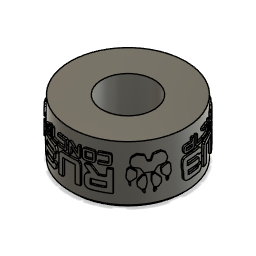
light v2 (Autodesk Fusion 360 design; units mm, degrees)
Autodesk Fusion 360 part; units mm, degrees
sketch "Esquisse1" plane through (0, 0, 0) normal (0, 1, 0) x (1, 0, 0)
  line L0 (25, 200) -> (-25, 200)
  line L1 (-25, 200) -> (-25, -200)
  line L2 (-25, -200) -> (25, -200)
  line L3 (25, -200) -> (25, 200)
  line L4 (25, 200) -> (-25, -200) construction
  line L5 (-25, 200) -> (25, -200) construction
  circle A0 centre (0, 100) radius 6.5
  circle A1 centre (0, 100) radius 4
  dimension "d1" = 50
  dimension "d2" = 400
  dimension "d3" = 13
  dimension "d4" = 8
  constraint horizontal L0
  constraint perpendicular L0 L1
  constraint parallel L0 L2
  constraint parallel L1 L3
  constraint coincident L4 origin
  constraint coincident L5 origin
  constraint concentric A0 A1
  measures "d1" distance of L1.end L2.end
  measures "d2" distance of L0.end L1.end
  measures "d3" diameter of A0
  measures "d4" diameter of A1
extrude "Extrusion1" add sketch "Esquisse1" against normal blind 6 contours L0 L1 L2 L3 makes body 1
extrude "Extrusion2" add sketch "Esquisse1" against normal blind 7 contours A0 bodies 1
fillet "Congé1" radius 3 1 edges at (-6.0601, -7, -102.3505) on bodies 1
extrude "Extrusion3" add 1 faces at (0.1619, -6, 102.1606) along direction (0, -1, 0) blind 9 and the other way blind -3 on bodies 1 bodies 1 makes body 2
extrude "Extrusion4" add sketch "Esquisse1" along normal blind -15 and the other way blind 8 contours A0 bodies 2
fillet "Congé2" radius 3 1 edges at (-6.0601, -8, -102.3505) on bodies 2
extrude "Extrusion5" add 1 faces at (0, -15, 101.3333) along direction (0, -1, 0) blind 6.5 and the other way blind -0.5 separate body on bodies 2 makes body 3
extrude "Extrusion6" add sketch "Esquisse1" along normal blind -22.5 and the other way blind 15.5 contours A0 bodies 3
fillet "Congé3" radius 3 1 edges at (-6.0601, -22.5, -102.3505) on bodies 3
extrude "Extrusion7" add sketch "Esquisse1" along normal blind 1 contours A0 bodies 1
fillet "Congé4" radius 3 1 edges at (-6.0601, 1, -97.6495) on bodies 1
extrude "Extrusion8" cut 2 faces at (-8.3333, -17.5, 200) (-8.3333, -11, 200) along direction (0, 0, -1) blind 270 on bodies 2 3 bodies 2 3
extrude "Extrusion9" add 1 faces at (-0.0996, -15, -167.9963) along direction (0, -1, 0) blind 0.25 separate body on bodies 2 makes body 4
revolve "Révolution1" add 1 faces at (-8.3333, -11, -70) angle 180 about axis through (25, -15.25, -70) along (1, 0, 0) on bodies 2 bodies 2 3 4
extrude "Extrusion10" cut 1 faces at (-0.0996, -15.25, -167.9963) along direction (0, 1, 0) blind 0.25 on bodies 2 bodies 2
sketch "Esquisse2" plane through (0, 0, 0) normal (0, -1, 0) x (1, 0, 0)
  line L0 (25, -70) -> (-25, -70)
  line L1 (-25, -70) -> (-25, -200)
  line L2 (-25, -200) -> (25, -200)
  line L3 (25, -200) -> (25, -70)
  circle A0 centre (0, -100) radius 6.5
  circle A1 centre (0, -100) radius 10
  circle A2 centre (0, -100) radius 3.5
  circle A3 centre (0, -100) radius 6.5
  line L4 (25, 200) -> (25, -200)
  line L5 (25, -200) -> (-25, -200)
  line L6 (-25, -200) -> (-25, 200)
  line L7 (-25, 200) -> (25, 200)
  dimension "d42" = 7
  constraint concentric A0 A1
  constraint concentric A1 A2
  measures "d42" diameter of A2
extrude "Extrusion11" add sketch "Esquisse2" along normal blind -1 and the other way blind 4 separate body contours A0 A3 | A1 | A2 makes body 5
fillet "Congé5" radius 2 1 edges at (-9.3233, 4, -96.3838) on bodies 5
fillet "Congé6" radius 1 1 edges at (-9.3233, 1, -96.3838) on bodies 5
extrude "Extrusion12" add sketch "Esquisse2" along normal blind 22.5 and the other way blind 1 contours A2 bodies 5
extrude "Extrusion13" add 1 faces at (1.7216, -22.5, -100.6592) along direction (0, -1, 0) blind 12 on bodies 5 bodies 5
ref_plane "Plan de construction1" through (0, 0, -100) normal (0, 0, 1) x (1, 0, 0)
sketch "Esquisse3" plane through (0, 0, -100) normal (0, 0, 1) x (1, 0, 0)
  line L0 (0, -32.5) -> (0, -22.5)
  line L1 (0, -22.5) -> (0, -22.7)
  circle A0 centre (0, -25.5) radius 1.7
  line L2 (0, -34.5) -> (-1.5, -34.5)
  line L3 (-1.5, -34.5) -> (-1.5, -32.5)
  circle A1 centre (-1.5, -32.5) radius 2
  circle A2 centre (1.5, -32.5) radius 2
  line L4 (3.5, -34.5) -> (3.5, -31.3)
  line L5 (-3.5, -34.5) -> (3.5, -34.5)
  line L6 (3.5, -34.5) -> (-3.5, -34.5)
  line L7 (-3.5, -34.5) -> (-3.5, -31.3)
  dimension "d60" = 3.4
  dimension "d65" = 1.5
  dimension "d66" = 2
  dimension "d67" = 4
  constraint vertical L0
  constraint coincident L0 L1.end
  constraint horizontal L2
  constraint perpendicular L2 L3
  constraint coincident L3.end A1.centre
  constraint symmetric L0 A1 A2
  constraint vertical L4
  constraint tangent A2 L4
  constraint coincident L4.start L5
  constraint coincident L4.start L5.end
  constraint coincident L5.start L6.end
  constraint perpendicular L6 L7
  constraint coincident L0 A0.centre
  measures "d60" diameter of A0
  measures "d65" distance of L2.start L2.end
  measures "d66" distance of L2.end L3.end
  measures "d67" diameter of A1
extrude "Extrusion14" cut sketch "Esquisse3" along normal blind 5 and the other way blind 5 contours L0 A0 | L0 A0 bodies 5
thread "Filetage2" "ISO Metric profile 7.0 M7x1 6g" major diameter 6.884 minor diameter 5.744 pitch 1 angle 60 modelled right hand crest width 0.1446 on face at (-2.0275, -19.6639, -102.8529) crest through (3.442, 1.25, -100) on bodies 5
revolve "Révolution2" cut sketch "Esquisse3" angle 360 about axis through (0, -32.5, -100) along (0, 1, 0) contours A1 L5 L6 L7 | A2 L4 L5 L6 bodies 5
sketch "Esquisse5" plane through (0, -34.5, 0) normal (0, -1, 0) x (1, 0, 0)
  circle A0 centre (0, -100) radius 1.5
  circle A1 centre (0, -100) radius 10
  circle A2 centre (0, -100) radius 3.5
  circle A3 centre (0, -100) radius 5.5
  circle A4 centre (0, -100) radius 9
  circle A5 centre (0, -100) radius 8.9
  line L0 (0, -108.9) -> (7.7076, -104.45)
  line L1 (7.7076, -104.45) -> (7.7076, -95.55)
  line L2 (7.7076, -95.55) -> (0, -91.1)
  line L3 (0, -91.1) -> (-7.7076, -95.55)
  line L4 (-7.7076, -95.55) -> (-7.7076, -104.45)
  line L5 (-7.7076, -104.45) -> (0, -108.9)
  line L6 (0, -109) -> (7.7942, -104.5)
  line L7 (7.7942, -104.5) -> (7.7942, -95.5)
  line L8 (7.7942, -95.5) -> (0, -91)
  line L9 (0, -91) -> (-7.7942, -95.5)
  line L10 (-7.7942, -95.5) -> (-7.7942, -104.5)
  line L11 (-7.7942, -104.5) -> (0, -109)
  point P0 (0, -100)
  point P1 (0, -100)
  dimension "d69" = 20
  dimension "d70" = 7
  dimension "d71" = 11
  dimension "d94" = -1
  dimension "d95" = -1.1
  constraint concentric A0 A1
  constraint concentric A1 A2
  constraint concentric A1 A3
  constraint coincident P1 P0
  constraint coincident A5 L0.start
  constraint coincident A4 L6.start
  measures "d69" diameter of A1
  measures "d70" diameter of A2
  measures "d71" diameter of A3
extrude "Extrusion16" add sketch "Esquisse5" against normal blind 7 separate body contours A2 | A3 | L0 L1 L2 L3 L4 L5 makes body 6
extrude "Extrusion19" add sketch "Esquisse5" against normal blind 7 separate body contours A0 | A1 | A2 | A3 | A4 A5 L7 | A4 A5 L8 | A5 L7 L8 | A4 A5 L6 | A5 L6 L7 | A4 A5 L9 | A5 L8 L9 | A5 L1 L7 | A5 L7 | A5 L8 | A5 L2 L8 | A5 L6 L11 | A4 A5 L11 | A5 L0 L6 | A5 L6 | A4 A5 L10 | A5 L9 L10 | A5 L9 | A5 L3 L9 | L0 L1 L2 L3 L4 L5 | A5 L10 L11 | A5 L5 L11 | A5 L11 | A5 L10 | A5 L4 L10 makes body 7
extrude "Extrusion18" add sketch "Esquisse5" along normal blind 3 contours A0 | A1 | A2 | A3 | A4 A5 L7 | A4 A5 L8 | A5 L7 L8 | A4 A5 L6 | A5 L6 L7 | A4 A5 L9 | A5 L8 L9 | A5 L1 L7 | A5 L7 | A5 L8 | A5 L2 L8 | A5 L6 L11 | A4 A5 L11 | A5 L0 L6 | A5 L6 | A4 A5 L10 | A5 L9 L10 | A5 L9 | A5 L3 L9 | L0 L1 L2 L3 L4 L5 | A5 L10 L11 | A5 L5 L11 | A5 L11 | A5 L10 | A5 L4 L10 bodies 7
chamfer "Chanfrein1" distance 0.5 angle 45 1 edges at (-9.3233, -37.5, -103.6162) on bodies 7
thread "Filetage4" "ISO Metric profile 7.0 M7x1 6H" major diameter 7.1472 minor diameter 6.0355 pitch 1 angle 60 modelled right hand crest width 0.2748 on face at (-1.3822, -29.8333, -99.4173) crest through (3.0178, -34.25, -100) on bodies 6
sketch "Esquisse8" plane through (0, -37.5, 0) normal (0, -1, 0) x (1, 0, 0)
  circle A0 centre (0, -100) radius 9.5
  line L0 (2.9064, -104.5301) -> (-0.138, -104.5283)
  line L1 (-0.1715, -103.4006) -> (6.1362, -103.4173)
  line L2 (-0.1498, -91.2683) -> (0.7478, -91.2683)
  line L3 (-3.1825, -104.5265) -> (-3.4574, -104.8217)
  line L4 (-7.2363, -105.0821) -> (-7.7542, -104.339)
  line L5 (0.7478, -91.2683) -> (1.3542, -92.1337)
  line L6 (3.194, -98.4202) -> (1.5775, -95.7423)
  line L7 (2.503, -93.8005) -> (3.0454, -94.6019)
  line L8 (1.5775, -95.7423) -> (-0.039, -93.0644)
  line L9 (-3.4574, -104.8217) -> (-3.7323, -105.1169)
  line L10 (-6.4792, -103.384) -> (-0.1715, -103.4006)
  line L11 (-3.3039, -98.1262) -> (-4.1512, -99.5305)
  line L12 (-4.8051, -98.2895) -> (-3.7281, -96.6567)
  line L13 (6.9426, -105.1148) -> (5.1818, -105.1148)
  line L14 (3.8431, -99.4978) -> (3.194, -98.4202)
  line L15 (4.2948, -97.9642) -> (5.5443, -99.857)
  line L16 (-0.138, -104.5283) -> (-3.1825, -104.5265)
  line L17 (1.3542, -92.1337) -> (1.9606, -92.9991)
  line L18 (7.9945, -103.5616) -> (7.4685, -104.3382)
  line L19 (-5.8821, -99.9224) -> (-4.8051, -98.2895)
  line L20 (3.0454, -94.6019) -> (3.0454, -95.3366)
  line L21 (-0.0703, -93.012) -> (-0.1016, -92.9596)
  line L22 (-0.1016, -92.9596) -> (-0.1579, -92.9794)
  line L23 (5.8501, -102.8229) -> (5.5109, -102.2816)
  line L24 (1.9606, -92.9991) -> (2.503, -93.8005)
  line L25 (-3.7323, -105.1169) -> (-5.4843, -105.0995)
  line L26 (3.0454, -95.3366) -> (3.0454, -96.0713)
  line L27 (-5.4843, -105.0995) -> (-7.2363, -105.0821)
  line L28 (6.7694, -101.7093) -> (7.9945, -103.5616)
  line L29 (3.0454, -96.0713) -> (4.2948, -97.9642)
  line L30 (-0.039, -93.0644) -> (-0.0703, -93.012)
  line L31 (5.1818, -105.1148) -> (3.4211, -105.1148)
  line L32 (-3.29, -95.244) -> (-3.29, -94.4979)
  line L33 (5.5443, -99.857) -> (6.7694, -101.7093)
  line L34 (4.852, -101.1633) -> (4.4923, -100.5755)
  line L35 (-3.29, -95.99) -> (-3.29, -95.244)
  line L36 (6.1894, -103.3641) -> (5.8501, -102.8229)
  line L37 (7.4685, -104.3382) -> (6.9426, -105.1148)
  line L38 (-4.1512, -99.5305) -> (-5.3152, -101.4572)
  line L39 (-8.2721, -103.5958) -> (-8.1528, -103.3919)
  line L40 (5.5109, -102.2816) -> (5.3614, -102.0164)
  line L41 (6.1628, -103.3907) -> (6.1894, -103.3641)
  line L42 (-1.3355, -94.8606) -> (-2.4567, -96.722)
  line L43 (-0.1579, -92.9794) -> (-0.2143, -92.9991)
  line L44 (4.4923, -100.5755) -> (3.8431, -99.4978)
  line L45 (-8.0335, -103.188) -> (-6.9578, -101.5552)
  line L46 (-3.7281, -96.6567) -> (-3.5091, -96.3234)
  line L47 (3.4211, -105.1148) -> (3.1638, -104.8224)
  line L48 (3.1638, -104.8224) -> (2.9064, -104.5301)
  line L49 (-1.0475, -91.2683) -> (-0.1498, -91.2683)
  line L50 (6.1362, -103.4173) -> (6.1628, -103.3907)
  line L51 (-2.4567, -96.722) -> (-3.3039, -98.1262)
  line L52 (-3.5091, -96.3234) -> (-3.29, -95.99)
  line L53 (5.3614, -102.0164) -> (5.2118, -101.7511)
  line L54 (-2.1687, -92.8831) -> (-1.0475, -91.2683)
  line L55 (-0.2143, -92.9991) -> (-1.3355, -94.8606)
  line L56 (5.2118, -101.7511) -> (4.852, -101.1633)
  line L57 (-5.3152, -101.4572) -> (-6.4792, -103.384)
  line L58 (-6.9578, -101.5552) -> (-5.8821, -99.9224)
  line L59 (-3.29, -94.4979) -> (-2.1687, -92.8831)
  line L60 (-8.1528, -103.3919) -> (-8.0335, -103.188)
  line L61 (-7.7542, -104.339) -> (-8.2721, -103.5958)
  line L62 (0.0351, -98.5913) -> (0.144, -98.2118)
  line L63 (0.144, -98.2118) -> (0.2529, -97.8323)
  line L64 (1.8612, -98.5508) -> (1.8237, -98.7141)
  line L65 (0.2892, -97.7909) -> (0.6713, -97.6996)
  line L66 (0.3736, -100.0203) -> (-0.1356, -100.0193)
  line L67 (1.1187, -97.6116) -> (1.184, -97.6149)
  line L68 (0.3736, -100.0203) -> (-0.1356, -100.0193)
  line L69 (1.4126, -97.776) -> (1.6412, -97.937)
  line L70 (1.6412, -97.937) -> (1.7512, -98.2439)
  line L71 (1.6412, -97.937) -> (1.7512, -98.2439)
  line L72 (1.1187, -97.6116) -> (1.184, -97.6149)
  line L73 (1.8612, -98.5508) -> (1.8237, -98.7141)
  line L74 (0.2711, -97.8116) -> (0.2892, -97.7909)
  line L75 (0.6288, -102.3571) -> (0.5003, -102.5113)
  line L76 (0.6713, -97.6996) -> (1.0533, -97.6084)
  line L77 (0.3697, -102.4533) -> (0.3675, -102.241)
  line L78 (-0.4833, -100.4515) -> (-0.4304, -100.8401)
  line L79 (0.3719, -102.6655) -> (0.3697, -102.4533)
  line L80 (0.2892, -97.7909) -> (0.6713, -97.6996)
  line L81 (-1.7781, -100.7657) -> (-2.0742, -101.0058)
  line L82 (2.239, -100.0641) -> (2.2789, -100.5812)
  line L83 (1.8237, -98.7141) -> (1.7861, -98.8773)
  line L84 (-1.9511, -99.1986) -> (-2.0658, -98.9726)
  line L85 (1.7512, -98.2439) -> (1.8612, -98.5508)
  line L86 (1.4698, -100.7535) -> (1.2055, -100.507)
  line L87 (0.1063, -100.8661) -> (0.1063, -100.4332)
  line L88 (-0.4916, -98.1974) -> (-0.3719, -98.5508)
  line L89 (0.144, -98.2118) -> (0.2529, -97.8323)
  line L90 (0.5003, -102.5113) -> (0.3719, -102.6655)
  line L91 (0.0351, -98.5913) -> (0.144, -98.2118)
  line L92 (-1.9511, -99.1986) -> (-2.0658, -98.9726)
  line L93 (-0.1684, -98.571) -> (0.0351, -98.5913)
  line L94 (1.7512, -98.2439) -> (1.8612, -98.5508)
  line L95 (1.8237, -98.7141) -> (1.7861, -98.8773)
  line L96 (-2.3363, -100.9674) -> (-2.4596, -100.7558)
  line L97 (1.4126, -97.776) -> (1.6412, -97.937)
  line L98 (-0.8457, -100.3469) -> (-0.7453, -100.3479)
  line L99 (-0.6113, -97.8441) -> (-0.4916, -98.1974)
  line L100 (-1.1347, -99.3697) -> (-1.2817, -99.3355)
  line L101 (1.184, -97.6149) -> (1.4126, -97.776)
  line L102 (-1.4649, -97.6044) -> (-1.0645, -97.6978)
  line L103 (-1.9781, -97.9284) -> (-1.7215, -97.7664)
  line L104 (-1.1347, -99.3697) -> (-1.2817, -99.3355)
  line L105 (1.0533, -97.6084) -> (1.1187, -97.6116)
  line L106 (-0.6642, -97.7912) -> (-0.6378, -97.8176)
  line L107 (-0.4506, -101.5917) -> (-0.5237, -101.9547)
  line L108 (-2.1144, -101.1307) -> (-2.1144, -101.3723)
  line L109 (-0.4916, -98.1974) -> (-0.3719, -98.5508)
  line L110 (1.184, -97.6149) -> (1.4126, -97.776)
  line L111 (0.2529, -97.8323) -> (0.2711, -97.8116)
  line L112 (-0.3719, -98.5508) -> (-0.1684, -98.571)
  line L113 (0.2529, -97.8323) -> (0.2711, -97.8116)
  line L114 (-2.1484, -98.4665) -> (-2.1161, -98.1863)
  line L115 (1.0533, -97.6084) -> (1.1187, -97.6116)
  line L116 (-0.3719, -98.5508) -> (-0.1684, -98.571)
  line L117 (0.6713, -97.6996) -> (1.0533, -97.6084)
  line L118 (0.2711, -97.8116) -> (0.2892, -97.7909)
  line L119 (0.4792, -100.2816) -> (0.8153, -100.6369)
  line L120 (-1.3091, -100.9021) -> (-1.0774, -100.6245)
  line L121 (-0.6378, -97.8176) -> (-0.6113, -97.8441)
  line L122 (-1.4649, -97.6044) -> (-1.0645, -97.6978)
  line L123 (-0.6378, -97.8176) -> (-0.6113, -97.8441)
  line L124 (-2.1806, -98.7467) -> (-2.1484, -98.4665)
  line L125 (-0.6448, -100.0183) -> (-0.7167, -99.9703)
  line L126 (-2.3245, -101.1307) -> (-2.2194, -101.1307)
  line L127 (0.6941, -99.4891) -> (0.5961, -99.6141)
  line L128 (0.439, -100.2816) -> (0.4591, -100.2816)
  line L129 (-2.49, -99.553) -> (-2.3552, -99.4275)
  line L130 (1.7341, -101) -> (1.4698, -100.7535)
  line L131 (-1.4202, -101.4208) -> (-1.4433, -101.1633)
  line L132 (0.4982, -102.241) -> (0.6288, -102.241)
  line L133 (0.7921, -99.364) -> (0.6941, -99.4891)
  line L134 (-2.2053, -100.9866) -> (-2.3363, -100.9674)
  line L135 (0.5961, -99.6141) -> (0.4849, -99.8172)
  line L136 (1.2055, -100.507) -> (1.1784, -100.1494)
  line L137 (0.2727, -100.3574) -> (0.439, -100.2816)
  line L138 (-2.1751, -101.5519) -> (-2.2357, -101.4899)
  line L139 (1.9111, -101.1287) -> (1.806, -101.1287)
  line L140 (1.806, -101.1287) -> (1.806, -101.3704)
  line L141 (2.2789, -100.5812) -> (2.1706, -100.7906)
  line L142 (-1.4686, -100.1537) -> (-1.482, -100.5256)
  line L143 (1.1784, -100.1494) -> (1.1513, -99.7917)
  line L144 (0.9777, -101.8241) -> (0.8042, -102.0517)
  line L145 (-1.798, -99.5418) -> (-1.4552, -99.7818)
  line L146 (-1.4286, -99.3013) -> (-1.6898, -99.25)
  line L147 (2.1706, -100.7906) -> (2.0623, -101)
  line L148 (1.1513, -100.9922) -> (1.1513, -101.2944)
  line L149 (0.1063, -100.4332) -> (0.2727, -100.3574)
  line L150 (-1.482, -100.5256) -> (-1.7781, -100.7657)
  line L151 (-0.1356, -100.0193) -> (-0.6448, -100.0183)
  line L152 (1.618, -99.2117) -> (1.205, -99.2879)
  line L153 (-0.7991, -102.1104) -> (-0.9784, -102.1104)
  line L154 (0.4849, -99.8172) -> (0.3736, -100.0203)
  line L155 (2.0834, -99.4592) -> (2.1992, -99.547)
  line L156 (1.9274, -101.4879) -> (1.9718, -101.3083)
  line L157 (-0.9617, -99.646) -> (-1.1347, -99.3697)
  line L158 (-1.4552, -99.7818) -> (-1.4686, -100.1537)
  line L159 (1.1513, -101.2944) -> (1.1513, -101.5966)
  line L160 (-2.2801, -101.3103) -> (-2.3245, -101.1307)
  line L161 (-2.1144, -101.614) -> (-2.1751, -101.5519)
  line L162 (1.806, -101.612) -> (1.8667, -101.55)
  line L163 (0.6941, -99.4891) -> (0.5961, -99.6141)
  line L164 (1.4772, -99.5795) -> (1.803, -99.3672)
  line L165 (2.1992, -99.547) -> (2.239, -100.0641)
  line L166 (-0.6122, -102.1757) -> (-0.6122, -102.4043)
  line L167 (-0.8029, -102.2364) -> (-0.7101, -102.1777)
  line L168 (-2.2204, -99.3019) -> (-2.1806, -99.3019)
  line L169 (-0.5718, -102.0325) -> (-0.6199, -102.1104)
  line L170 (-2.5828, -100.5441) -> (-2.5364, -100.0486)
  line L171 (-0.7851, -102.464) -> (-0.8957, -102.2952)
  line L172 (-0.6199, -102.1104) -> (-0.7991, -102.1104)
  line L173 (-1.4286, -99.3013) -> (-1.6898, -99.25)
  line L174 (0.3567, -102.0124) -> (0.2315, -101.6557)
  line L175 (1.618, -99.2117) -> (1.205, -99.2879)
  line L176 (-0.9784, -102.1104) -> (-1.1878, -101.8944)
  line L177 (0.2315, -101.6557) -> (0.1063, -101.299)
  line L178 (-2.1806, -99.3019) -> (-2.1408, -99.3019)
  line L179 (1.9718, -101.3083) -> (2.0161, -101.1287)
  line L180 (-0.6611, -102.1767) -> (-0.6122, -102.1757)
  line L181 (0.6288, -102.2991) -> (0.6288, -102.3571)
  line L182 (-1.2817, -99.3355) -> (-1.4286, -99.3013)
  line L183 (0.8042, -102.0517) -> (0.5804, -102.032)
  line L184 (0.3675, -102.241) -> (0.4982, -102.241)
  line L185 (-0.5237, -101.9547) -> (-0.5718, -102.0325)
  line L186 (-0.8957, -102.2952) -> (-0.8029, -102.2364)
  line L187 (1.8854, -99.3693) -> (1.9677, -99.3714)
  line L188 (-2.4596, -100.7558) -> (-2.5828, -100.5441)
  line L189 (-0.6122, -102.4043) -> (-0.6122, -102.6329)
  line L190 (-0.6433, -102.6329) -> (-0.6745, -102.6329)
  line L191 (-0.6122, -102.6329) -> (-0.6433, -102.6329)
  line L192 (-0.7101, -102.1777) -> (-0.6611, -102.1767)
  line L193 (-0.6745, -102.6329) -> (-0.7851, -102.464)
  line L194 (2.0623, -101) -> (1.8982, -101)
  line L195 (0.6288, -102.241) -> (0.6288, -102.2991)
  line L196 (-1.6898, -99.25) -> (-1.9511, -99.1986)
  line L197 (1.806, -101.3704) -> (1.806, -101.612)
  line L198 (0.5961, -99.6141) -> (0.4849, -99.8172)
  line L199 (-0.7167, -99.9703) -> (-0.7886, -99.9224)
  line L200 (-1.0774, -100.6245) -> (-0.8457, -100.3469)
  line L201 (0.4849, -99.8172) -> (0.3736, -100.0203)
  line L202 (1.1513, -99.7917) -> (1.4772, -99.5795)
  line L203 (-2.0658, -98.9726) -> (-2.1806, -98.7467)
  line L204 (-0.7886, -99.9224) -> (-0.9617, -99.646)
  line L205 (-1.2817, -99.3355) -> (-1.4286, -99.3013)
  line L206 (-1.7215, -97.7664) -> (-1.4649, -97.6044)
  line L207 (1.9677, -99.3714) -> (2.0834, -99.4592)
  line L208 (-2.1161, -98.1863) -> (-2.0471, -98.0573)
  line L209 (1.8982, -101) -> (1.7341, -101)
  line L210 (-1.6898, -99.25) -> (-1.9511, -99.1986)
  line L211 (-0.6448, -100.0183) -> (-0.7167, -99.9703)
  line L212 (-2.0471, -98.0573) -> (-1.9781, -97.9284)
  line L213 (0.7921, -99.364) -> (0.6941, -99.4891)
  line L214 (1.1513, -101.5966) -> (0.9777, -101.8241)
  line L215 (0.4591, -100.2816) -> (0.4792, -100.2816)
  line L216 (1.702, -99.0445) -> (1.618, -99.2117)
  line L217 (-2.2357, -101.4899) -> (-2.2801, -101.3103)
  line L218 (-2.0658, -98.9726) -> (-2.1806, -98.7467)
  line L219 (-2.0742, -101.0058) -> (-2.2053, -100.9866)
  line L220 (-0.4304, -100.8401) -> (-0.3776, -101.2286)
  line L221 (-2.5364, -100.0486) -> (-2.49, -99.553)
  line L222 (1.8667, -101.55) -> (1.9274, -101.4879)
  line L223 (1.7861, -98.8773) -> (1.702, -99.0445)
  line L224 (-0.1356, -100.0193) -> (-0.6448, -100.0183)
  line L225 (-2.1161, -98.1863) -> (-2.0471, -98.0573)
  line L226 (-1.4433, -101.1633) -> (-1.3762, -101.0327)
  line L227 (-0.9617, -99.646) -> (-1.1347, -99.3697)
  line L228 (-0.6113, -97.8441) -> (-0.4916, -98.1974)
  line L229 (-2.1484, -98.4665) -> (-2.1161, -98.1863)
  line L230 (-0.1684, -98.571) -> (0.0351, -98.5913)
  line L231 (0.8153, -100.6369) -> (1.1513, -100.9922)
  line L232 (1.7861, -98.8773) -> (1.702, -99.0445)
  line L233 (-2.1144, -101.3723) -> (-2.1144, -101.614)
  line L234 (-1.9781, -97.9284) -> (-1.7215, -97.7664)
  line L235 (-2.2194, -101.1307) -> (-2.1144, -101.1307)
  line L236 (-0.564, -100.4002) -> (-0.4833, -100.4515)
  line L237 (-1.0645, -97.6978) -> (-0.6642, -97.7912)
  line L238 (-2.0471, -98.0573) -> (-1.9781, -97.9284)
  line L239 (0.1063, -101.299) -> (0.1063, -100.8661)
  line L240 (-0.6642, -97.7912) -> (-0.6378, -97.8176)
  line L241 (-2.3552, -99.4275) -> (-2.2204, -99.3019)
  line L242 (1.702, -99.0445) -> (1.618, -99.2117)
  line L243 (-1.0645, -97.6978) -> (-0.6642, -97.7912)
  line L244 (-0.7453, -100.3479) -> (-0.6448, -100.3489)
  line L245 (-0.6448, -100.3489) -> (-0.564, -100.4002)
  line L246 (1.803, -99.3672) -> (1.8854, -99.3693)
  line L247 (-1.3971, -101.6784) -> (-1.4202, -101.4208)
  line L248 (1.205, -99.2879) -> (0.7921, -99.364)
  line L249 (-0.7886, -99.9224) -> (-0.9617, -99.646)
  line L250 (-0.3776, -101.2286) -> (-0.4506, -101.5917)
  line L251 (0.5804, -102.032) -> (0.3567, -102.0124)
  line L252 (-1.3762, -101.0327) -> (-1.3091, -100.9021)
  line L253 (2.0161, -101.1287) -> (1.9111, -101.1287)
  line L254 (-0.7167, -99.9703) -> (-0.7886, -99.9224)
  line L255 (-2.1806, -98.7467) -> (-2.1484, -98.4665)
  line L256 (-2.1408, -99.3019) -> (-1.798, -99.5418)
  line L257 (-1.1878, -101.8944) -> (-1.3971, -101.6784)
  line L258 (1.205, -99.2879) -> (0.7921, -99.364)
  line L259 (-1.7215, -97.7664) -> (-1.4649, -97.6044)
  circle A1 centre (0, -100) radius 9.5
emboss "Gravure en relief2" depth -0.4 profiles "Esquisse8" section 1 contours L0 L2 L3 L4 L5 L7 L9 L12 L13 L15 L16 L17 L18 L19 L20 L24 L25 L26 L27 L28 L29 L31 L32 L33 L35 L37 L39 L45 L46 L47 L48 L49 L52 L54 L58 L59 L60 L61 | L62 L63 L64 L65 L66 L67 L68 L69 L70 L71 L72 L73 L74 L76 L80 L83 L84 L85 L88 L89 L91 L92 L93 L94 L95 L97 L99 L100 L101 L102 L103 L104 L105 L106 L109 L110 L111 L112 L113 L114 L115 L116 L117 L118 L121 L122 L123 L124 L125 L127 L133 L135 L146 L151 L152 L154 L157 L163 L173 L175 L182 L196 L198 L199 L201 L203 L204 L205 L206 L208 L210 L211 L212 L213 L216 L218 L223 L224 L225 L227 L228 L229 L230 L232 L234 L237 L238 L240 L242 L243 L248 L249 L254 L255 L258 L259 | L75 L77 L79 L90 L132 L181 L184 L195 | L78 L98 L107 L120 L131 L153 L169 L172 L176 L185 L200 L220 L226 L236 L244 L245 L247 L250 L252 L257 | L81 L96 L129 L134 L142 L145 L150 L158 L168 L170 L178 L188 L219 L221 L241 L256 | L82 L86 L130 L136 L141 L143 L147 L155 L164 L165 L187 L194 L202 L207 L209 L246 | L87 L119 L128 L137 L144 L148 L149 L159 L174 L177 L183 L214 L215 L231 L239 L251 | L108 L126 L138 L160 L161 L217 L233 L235 | L139 L140 L156 L162 L179 L197 L222 L253 | L166 L167 L171 L180 L186 L189 L190 L191 L192 L193 onto face at (-0.0584, -37.5, -92.9045) on bodies 7 bodies 7
sketch "Esquisse9" plane through (0, 0, 0) normal (0, 0, 1) x (1, 0, 0)
  line L0 (12.0165, -32.6685) -> (11.985, -32.2529)
  line L1 (7.6146, -32.7116) -> (7.6686, -32.1358)
  line L2 (8.9249, -31.8259) -> (8.9093, -32.258)
  line L3 (9.633, -32.4825) -> (9.7498, -32.4836)
  line L4 (13.2174, -32.1538) -> (13.2638, -32.7547)
  line L5 (-5.2181, -32.6758) -> (-5.2181, -33.03)
  spline S0 degree 3 poles (4.9372, -29.2993) (5.6787, -29.2993) (5.6974, -29.3018) (5.8108, -29.4152) knots 0 0 0 0 1 1 1 1
  line L6 (-4.9914, -29.9028) -> (-4.3917, -29.8896)
  line L7 (-4.1792, -32.3216) -> (-5.2181, -32.3216)
  line L8 (0.775, -30.3182) -> (0.4252, -29.8967)
  line L9 (0.0238, -31.0995) -> (0.0238, -30.1994)
  line L10 (-5.3978, -30.4917) -> (-5.4121, -30.716)
  line L11 (-4.3917, -29.8896) -> (-4.3776, -29.5945)
  line L12 (2.4794, -30.1966) -> (2.4794, -30.716)
  spline S1 degree 3 poles (-5.6709, -30.9377) (-5.8268, -30.7563) (-5.8368, -30.2283) (-5.688, -30.0391) knots 0 0 0 0 1 1 1 1
  line L13 (-3.4944, -29.2993) -> (-3.3291, -29.2993)
  line L14 (-2.0541, -30.9081) -> (-2.0541, -30.716)
  spline S2 degree 3 poles (3.8127, -29.4606) (3.8318, -29.4888) (3.8478, -29.822) (3.8482, -30.2011) knots 0 0 0 0 1 1 1 1
  line L15 (-5.557, -31.0702) -> (-5.6709, -30.9377)
  line L16 (-4.1759, -29.2993) -> (-3.9882, -29.2993)
  line L17 (0.4015, -30.4835) -> (0.3779, -31.0702)
  line L18 (-1.0638, -35.2023) -> (-1.4427, -35.2023)
  line L19 (-2.9986, -33.4078) -> (-2.9986, -33.7856)
  spline S3 degree 3 poles (-2.8033, -31.0938) (-3.3464, -31.0938) (-3.424, -31.0835) (-3.5353, -30.996) knots 0 0 0 0 1 1 1 1
  line L20 (-3.6597, -29.2993) -> (-3.4944, -29.2993)
  line L21 (3.5183, -30.1966) -> (3.5183, -29.6771)
  line L22 (5.5489, -30.716) -> (5.5489, -30.1966)
  spline S4 degree 3 poles (3.8482, -30.2011) (3.8491, -31.0902) (3.8717, -31.064) (3.0842, -31.0861) knots 0 0 0 0 1 1 1 1
  line L23 (4.8642, -30.716) -> (5.5489, -30.716)
  line L24 (-5.4121, -30.716) -> (-4.8901, -30.716)
  line L25 (-5.2181, -33.03) -> (-4.1083, -33.03)
  line L26 (-1.8216, -35.2023) -> (-1.808, -33.6237)
  line L27 (-2.7624, -34.1634) -> (-2.3847, -34.1634)
  line L28 (-5.0764, -34.1161) -> (-5.0764, -34.4467)
  line L29 (-2.6465, -35.0155) -> (-2.8148, -35.1787)
  line L30 (-3.1402, -34.4467) -> (-3.1402, -34.305)
  spline S5 degree 3 poles (5.8108, -29.4152) (5.9228, -29.5273) (5.9267, -29.553) (5.9252, -30.1826) knots 0 0 0 0 1 1 1 1
  line L31 (0.2008, -31.0849) -> (0.0238, -31.0995)
  spline S6 degree 3 poles (-5.688, -30.0391) (-5.5939, -29.9195) (-5.5743, -29.9157) (-4.9914, -29.9028) knots 0 0 0 0 1 1 1 1
  line L32 (4.1794, -30.716) -> (4.8642, -30.716)
  line L33 (6.0684, -35.2023) -> (4.4934, -35.2023)
  spline S7 degree 3 poles (-0.4312, -29.3972) (-0.3068, -29.4951) (-0.3068, -29.4953) (-0.3068, -30.1927) knots 0 0 0 0 1 1 1 1
  line L34 (-2.0541, -29.4882) -> (-2.0541, -29.2993)
  line L35 (-2.1958, -30.9049) -> (-2.1958, -31.0938)
  line L36 (-5.0764, -34.4467) -> (-4.1083, -34.4467)
  line L37 (-4.8757, -30.254) -> (-5.3834, -30.2674)
  line L38 (-4.3635, -29.2993) -> (-4.1759, -29.2993)
  spline S8 degree 3 poles (-5.8319, -34.1116) (-5.832, -33.6644) (-5.8506, -33.4796) (-5.9066, -33.3672) knots 0 0 0 0 1 1 1 1
  line L39 (-2.3847, -34.1634) -> (-2.385, -34.3404)
  line L40 (-1.4427, -35.2023) -> (-1.8216, -35.2023)
  spline S9 degree 3 poles (-5.4901, -35.1093) (-5.7801, -34.9302) (-5.8317, -34.7796) (-5.8319, -34.1116) knots 0 0 0 0 1 1 1 1
  spline S10 degree 3 poles (-5.8523, -31.8645) (-5.6448, -31.582) (-5.5559, -31.5662) (-4.1744, -31.5661) knots 0 0 0 0 1 1 1 1
  line L41 (4.2267, -33.5494) -> (3.1877, -33.5494)
  line L42 (-3.3291, -29.2993) -> (-3.3291, -30.0077)
  line L43 (-2.0541, -29.6771) -> (-2.0541, -29.4882)
  line L44 (-4.3776, -29.5945) -> (-4.3635, -29.2993)
  line L45 (4.2284, -32.7939) -> (4.7249, -32.7939)
  line L46 (-4.368, -30.4783) -> (-4.368, -30.2406)
  line L47 (-3.5353, -30.996) -> (-3.6597, -30.8981)
  line L48 (3.5183, -30.716) -> (3.5183, -30.1966)
  line L49 (1.4301, -29.9005) -> (1.4433, -29.2993)
  line L50 (-1.0513, -33.7738) -> (-1.0638, -35.2023)
  spline S11 degree 3 poles (1.6153, -31.0938) (1.4394, -31.0938) (1.3515, -31.0127) (0.775, -30.3182) knots 0 0 0 0 1 1 1 1
  line L51 (5.2892, -31.5897) -> (5.6788, -31.5759)
  line L52 (-4.7854, -31.0702) -> (-5.557, -31.0702)
  spline S12 degree 3 poles (4.7249, -32.7939) (5.1119, -32.7939) (5.227, -32.779) (5.2473, -32.7263) knots 0 0 0 0 1 1 1 1
  line L53 (3.5183, -29.6771) -> (2.9989, -29.6771)
  line L54 (3.1877, -34.4467) -> (4.2267, -34.4467)
  line L55 (-3.6597, -30.8981) -> (-3.6597, -30.0987)
  line L56 (4.1794, -30.9049) -> (4.1794, -30.716)
  spline S13 degree 3 poles (3.6836, -29.3558) (3.7355, -29.3852) (3.7937, -29.4324) (3.8127, -29.4606) knots 0 0 0 0 1 1 1 1
  line L57 (-4.001, -30.1848) -> (-4.0139, -31.0702)
  line L58 (-2.0541, -31.1002) -> (-2.0541, -30.9081)
  line L59 (4.1794, -29.4882) -> (4.1794, -29.2993)
  line L60 (0.3779, -31.0702) -> (0.2008, -31.0849)
  line L61 (4.1794, -29.6771) -> (4.1794, -29.4882)
  spline S14 degree 3 poles (0.209, -29.2993) (0.388, -29.2993) (0.4114, -29.3195) (0.9056, -29.9005) knots 0 0 0 0 1 1 1 1
  spline S15 degree 3 poles (5.9252, -30.1826) (5.9231, -31.0949) (5.9243, -31.0938) (4.8909, -31.0938) knots 0 0 0 0 1 1 1 1
  spline S16 degree 3 poles (-5.9656, -32.6077) (-5.9522, -32.0799) (-5.9369, -31.9797) (-5.8523, -31.8645) knots 0 0 0 0 1 1 1 1
  line L62 (4.8642, -29.6771) -> (4.1794, -29.6771)
  line L63 (4.8909, -31.0938) -> (4.1794, -31.0938)
  line L64 (0.0238, -30.1994) -> (0.0238, -29.2993)
  line L65 (5.5489, -29.6771) -> (4.8642, -29.6771)
  line L66 (4.1794, -31.0938) -> (4.1794, -30.9049)
  line L67 (0.0238, -29.2993) -> (0.209, -29.2993)
  line L68 (5.5489, -30.1966) -> (5.5489, -29.6771)
  line L69 (0.4252, -29.8967) -> (0.4015, -30.4835)
  line L70 (-0.6374, -30.1966) -> (-0.6374, -29.6771)
  line L71 (12.3322, -31.5907) -> (12.7108, -31.3441)
  line L72 (5.2812, -32.1242) -> (5.2892, -31.5897)
  spline S17 degree 3 poles (5.2715, -34.0925) (5.2715, -33.9497) (5.2702, -33.769) (5.2685, -33.6911) knots 0 0 0 0 1 1 1 1
  line L73 (9.8747, -29.5435) -> (9.9054, -29.5743)
  line L74 (10.8847, -34.0032) -> (10.7393, -33.5887)
  line L75 (-2.1958, -31.0938) -> (-2.8033, -31.0938)
  spline S18 degree 3 poles (4.2267, -34.4467) (4.8858, -34.4467) (5.2667, -34.4294) (5.2685, -34.3995) knots 0 0 0 0 1 1 1 1
  line L76 (11.1792, -31.867) -> (11.0499, -32.103)
  line L77 (12.8553, -33.8083) -> (12.9069, -33.5996)
  line L78 (11.3477, -34.8167) -> (11.1971, -34.9975)
  line L79 (8.2153, -30.8856) -> (8.082, -30.6231)
  line L80 (-1.3457, -29.6771) -> (-2.0541, -29.6771)
  line L81 (5.2656, -33.5494) -> (4.2267, -33.5494)
  line L82 (12.7784, -30.3954) -> (12.7348, -30.5852)
  spline S19 degree 3 poles (2.9613, -29.3008) (3.3397, -29.3016) (3.6267, -29.3235) (3.6836, -29.3558) knots 0 0 0 0 1 1 1 1
  line L83 (11.3085, -31.631) -> (11.1792, -31.867)
  line L84 (12.7143, -33.3909) -> (12.7143, -33.6717)
  line L85 (-2.3714, -32.5577) -> (-2.7558, -32.5577)
  line L86 (2.4794, -30.716) -> (2.9989, -30.716)
  line L87 (9.3788, -29.4043) -> (9.844, -29.5128)
  line L88 (12.5935, -30.9692) -> (12.4958, -31.1635)
  line L89 (11.8397, -29.3004) -> (11.9156, -29.3042)
  line L90 (11.0302, -34.4177) -> (10.8847, -34.0032)
  line L91 (8.9558, -31.2675) -> (8.6522, -31.2079)
  line L92 (9.1265, -31.3072) -> (8.9558, -31.2675)
  line L93 (8.3172, -29.6722) -> (8.6154, -29.484)
  line L94 (12.7143, -33.6717) -> (12.7143, -33.9525)
  line L95 (12.6506, -30.0389) -> (12.7784, -30.3954)
  line L96 (-0.6374, -30.716) -> (-0.6374, -30.1966)
  line L97 (13.1711, -31.553) -> (13.2174, -32.1538)
  line L98 (-2.1958, -30.716) -> (-2.1958, -30.9049)
  spline S20 degree 3 poles (5.2685, -34.3995) (5.2702, -34.3735) (5.2715, -34.2354) (5.2715, -34.0925) knots 0 0 0 0 1 1 1 1
  line L99 (-3.1402, -32.3216) -> (-4.1792, -32.3216)
  line L100 (12.6911, -30.7749) -> (12.5935, -30.9692)
  spline S21 degree 3 poles (-1.3049, -29.2993) (-0.6184, -29.2993) (-0.5452, -29.3075) (-0.4312, -29.3972) knots 0 0 0 0 1 1 1 1
  line L101 (11.9156, -29.3042) -> (11.9915, -29.308)
  line L102 (12.7143, -33.9525) -> (12.7848, -33.8804)
  line L103 (3.7218, -32.18) -> (4.2284, -32.7939)
  line L104 (9.783, -32.0449) -> (9.6995, -31.9892)
  line L105 (8.3487, -31.1482) -> (8.2153, -30.8856)
  line L106 (-2.3992, -32.289) -> (-2.3714, -32.5577)
  line L107 (-4.1083, -34.4467) -> (-3.1402, -34.4467)
  line L108 (-2.8148, -35.1787) -> (-4.0755, -35.1915)
  line L109 (7.6686, -32.1358) -> (7.7225, -31.56)
  line L110 (13.0366, -31.4509) -> (13.1711, -31.553)
  line L111 (10.7831, -30.0016) -> (10.9096, -29.5606)
  line L112 (-2.0541, -30.716) -> (-1.3457, -30.716)
  spline S22 degree 3 poles (-2.762, -31.6723) (-2.5228, -31.835) (-2.4297, -31.9934) (-2.3992, -32.289) knots 0 0 0 0 1 1 1 1
  line L113 (8.082, -31.2682) -> (8.1282, -31.2682)
  line L114 (8.6522, -31.2079) -> (8.3487, -31.1482)
  line L115 (-4.0139, -31.0702) -> (-4.7854, -31.0702)
  spline S23 degree 3 poles (2.1948, -30.951) (2.1109, -30.867) (2.1016, -30.7919) (2.1016, -30.1944) knots 0 0 0 0 1 1 1 1
  line L116 (12.2571, -29.4952) -> (12.5227, -29.6823)
  line L117 (12.7848, -33.8804) -> (12.8553, -33.8083)
  spline S24 degree 3 poles (2.1016, -30.1944) (2.1016, -29.5532) (2.1054, -29.5273) (2.2175, -29.4152) knots 0 0 0 0 1 1 1 1
  line L118 (-2.0541, -29.2993) -> (-1.3049, -29.2993)
  line L119 (11.1971, -34.9975) -> (11.0479, -35.1766)
  line L120 (10.6565, -30.4425) -> (10.7831, -30.0016)
  line L121 (-4.8901, -30.716) -> (-4.368, -30.716)
  line L122 (11.0479, -35.1766) -> (11.0453, -34.93)
  line L123 (11.9535, -33.9345) -> (11.7518, -34.199)
  spline S25 degree 3 poles (-1.808, -33.6237) (-1.7949, -32.1071) (-1.7905, -32.0398) (-1.6956, -31.9118) knots 0 0 0 0 1 1 1 1
  line L124 (-3.1402, -34.1634) -> (-2.7624, -34.1634)
  line L125 (11.7518, -34.199) -> (11.5502, -34.4634)
  line L126 (11.3958, -29.4065) -> (11.8397, -29.3004)
  line L127 (2.4794, -29.6771) -> (2.4794, -30.1966)
  line L128 (11.5502, -34.4634) -> (11.2902, -34.4405)
  line L129 (-5.3834, -30.2674) -> (-5.3978, -30.4917)
  line L130 (6.0684, -33.3823) -> (6.0684, -35.2023)
  line L131 (11.3464, -34.7508) -> (11.3477, -34.8167)
  line L132 (-2.7624, -30.716) -> (-2.1958, -30.716)
  line L133 (10.9307, -29.5366) -> (10.9518, -29.5125)
  line L134 (12.7108, -31.3441) -> (12.8065, -31.3465)
  spline S26 degree 3 poles (2.2175, -29.4152) (2.3291, -29.3036) (2.3567, -29.2994) (2.9613, -29.3008) knots 0 0 0 0 1 1 1 1
  line L135 (-3.9882, -29.2993) -> (-4.001, -30.1848)
  spline S27 degree 3 poles (5.2473, -32.7263) (5.2615, -32.6891) (5.2768, -32.4182) (5.2812, -32.1242) knots 0 0 0 0 1 1 1 1
  line L136 (11.5361, -31.3403) -> (11.4223, -31.4857)
  line L137 (1.4433, -29.2993) -> (1.6072, -29.2993)
  line L138 (-3.6597, -30.0987) -> (-3.6597, -29.2993)
  line L139 (-5.2181, -32.3216) -> (-5.2181, -32.6758)
  line L140 (1.771, -31.0938) -> (1.6153, -31.0938)
  line L141 (11.0453, -34.93) -> (11.0428, -34.6833)
  line L142 (11.0499, -32.103) -> (10.4582, -32.1018)
  line L143 (-1.0388, -32.3452) -> (-1.0513, -33.7738)
  line L144 (11.0428, -34.6833) -> (11.1946, -34.6833)
  line L145 (-1.2797, -31.0852) -> (-2.0541, -31.1002)
  line L146 (11.9535, -31.8374) -> (12.3322, -31.5907)
  line L147 (11.2902, -34.4405) -> (11.0302, -34.4177)
  line L148 (-5.0764, -33.7856) -> (-5.0764, -34.1161)
  spline S28 degree 3 poles (-0.3068, -30.1927) (-0.3068, -31.116) (-0.2515, -31.0653) (-1.2797, -31.0852) knots 0 0 0 0 1 1 1 1
  line L149 (-3.1402, -34.305) -> (-3.1402, -34.1634)
  line L150 (-4.0375, -33.7856) -> (-5.0764, -33.7856)
  spline S29 degree 3 poles (-5.9066, -33.3672) (-5.9659, -33.2485) (-5.978, -33.0923) (-5.9656, -32.6077) knots 0 0 0 0 1 1 1 1
  spline S30 degree 3 poles (-4.0755, -35.1915) (-5.2687, -35.2037) (-5.3444, -35.1993) (-5.4901, -35.1093) knots 0 0 0 0 1 1 1 1
  line L151 (6.0684, -31.5622) -> (6.0684, -33.3823)
  line L152 (-0.6374, -29.6771) -> (-1.3457, -29.6771)
  line L153 (11.1946, -34.6833) -> (11.3464, -34.6833)
  line L154 (4.1794, -29.2993) -> (4.9372, -29.2993)
  line L155 (10.9096, -29.5606) -> (10.9307, -29.5366)
  line L156 (5.6788, -31.5759) -> (6.0684, -31.5622)
  line L157 (-4.368, -30.716) -> (-4.368, -30.4783)
  line L158 (11.3464, -34.6833) -> (11.3464, -34.7508)
  line L159 (3.2153, -31.5661) -> (3.7218, -32.18)
  line L160 (-4.368, -30.2406) -> (-4.8757, -30.254)
  spline S31 degree 3 poles (-2.385, -34.3404) (-2.3854, -34.6295) (-2.4678, -34.8422) (-2.6465, -35.0155) knots 0 0 0 0 1 1 1 1
  line L161 (12.016, -31.2519) -> (11.5361, -31.3403)
  line L162 (12.8065, -31.3465) -> (12.9022, -31.3489)
  line L163 (5.2685, -33.6911) -> (5.2656, -33.5494)
  line L164 (12.7348, -30.5852) -> (12.6911, -30.7749)
  line L165 (1.4169, -30.5016) -> (1.4301, -29.9005)
  line L166 (-3.3291, -30.0077) -> (-3.3291, -30.716)
  line L167 (2.9989, -30.716) -> (3.5183, -30.716)
  line L168 (1.771, -29.2993) -> (1.771, -30.1966)
  line L169 (8.9093, -32.258) -> (8.8937, -32.6901)
  line L170 (9.3638, -32.805) -> (9.633, -32.4825)
  line L171 (9.9604, -32.5444) -> (10.0542, -32.604)
  line L172 (7.9148, -33.3932) -> (8.0369, -33.3932)
  line L173 (9.0167, -33.2793) -> (9.0947, -33.1275)
  line L174 (8.8937, -32.6901) -> (8.5496, -32.9691)
  line L175 (7.7578, -32.9575) -> (7.6146, -32.7116)
  line L176 (7.9664, -33.6019) -> (7.9148, -33.3932)
  spline S32 degree 3 poles (2.3923, -34.1226) (2.3829, -33.777) (2.3981, -33.4398) (2.4281, -33.3283) knots 0 0 0 0 1 1 1 1
  line L177 (1.4405, -35.2023) -> (1.0627, -35.2023)
  line L178 (3.1877, -33.5494) -> (3.1877, -33.9981)
  line L179 (8.0533, -33.2258) -> (7.901, -33.2034)
  line L180 (10.0542, -32.604) -> (10.1156, -33.0555)
  spline S33 degree 3 poles (-0.0047, -31.5661) (1.1196, -31.5662) (1.2952, -31.5762) (1.4395, -31.6488) knots 0 0 0 0 1 1 1 1
  spline S34 degree 3 poles (1.7111, -31.8918) (1.8172, -32.0506) (1.8183, -32.0684) (1.8183, -33.6273) knots 0 0 0 0 1 1 1 1
  spline S35 degree 3 poles (1.4395, -31.6488) (1.5299, -31.6942) (1.6521, -31.8035) (1.7111, -31.8918) knots 0 0 0 0 1 1 1 1
  line L181 (10.1156, -33.0555) -> (10.177, -33.507)
  line L182 (9.7498, -32.4836) -> (9.8665, -32.4848)
  line L183 (1.0627, -35.2023) -> (1.0627, -33.761)
  line L184 (8.2056, -33.2481) -> (8.0533, -33.2258)
  line L185 (7.901, -33.2034) -> (7.7578, -32.9575)
  line L186 (8.5496, -32.9691) -> (8.2056, -33.2481)
  line L187 (9.8665, -32.4848) -> (9.9604, -32.5444)
  line L188 (11.1259, -32.4066) -> (11.1492, -32.4066)
  line L189 (-3.3291, -30.716) -> (-2.7624, -30.716)
  line L190 (-2.9986, -33.03) -> (-2.9986, -33.4078)
  line L191 (12.9584, -33.3909) -> (12.8364, -33.3909)
  line L192 (9.2972, -31.347) -> (9.1265, -31.3072)
  line L193 (9.8665, -32.1007) -> (9.783, -32.0449)
  line L194 (1.6072, -29.2993) -> (1.771, -29.2993)
  line L195 (9.9045, -35.1387) -> (9.8683, -35.1387)
  line L196 (9.6872, -34.5315) -> (9.4789, -34.5315)
  line L197 (8.082, -30.6231) -> (8.1194, -30.2975)
  line L198 (12.9022, -31.3489) -> (13.0366, -31.4509)
  line L199 (13.1379, -32.9981) -> (13.0121, -33.2414)
  line L200 (9.5749, -34.7463) -> (9.6828, -34.678)
  line L201 (11.985, -32.2529) -> (11.9535, -31.8374)
  line L202 (11.9915, -29.308) -> (12.2571, -29.4952)
  spline S36 degree 3 poles (2.4281, -33.3283) (2.4942, -33.0831) (2.7989, -32.7939) (2.9911, -32.7939) knots 0 0 0 0 1 1 1 1
  line L203 (7.7225, -31.56) -> (7.8792, -31.4141)
  line L204 (2.9989, -29.6771) -> (2.4794, -29.6771)
  line L205 (12.9069, -33.5996) -> (12.9584, -33.3909)
  line L206 (8.9136, -29.2958) -> (9.3788, -29.4043)
  line L207 (0.9056, -29.9005) -> (1.4169, -30.5016)
  line L208 (9.9045, -34.8731) -> (9.9045, -35.1387)
  line L209 (12.6307, -33.2414) -> (12.3236, -32.9549)
  line L210 (1.771, -30.1966) -> (1.771, -31.0938)
  line L211 (11.4223, -31.4857) -> (11.3085, -31.631)
  line L212 (8.0358, -31.2682) -> (8.082, -31.2682)
  line L213 (-1.3457, -30.716) -> (-0.6374, -30.716)
  line L214 (8.6154, -29.484) -> (8.9136, -29.2958)
  line L215 (9.9045, -34.6074) -> (9.9045, -34.8731)
  line L216 (9.7906, -34.6098) -> (9.8475, -34.6086)
  line L217 (12.8214, -33.2414) -> (12.6307, -33.2414)
  line L218 (-3.1402, -32.4397) -> (-3.1402, -32.3216)
  line L219 (8.5266, -31.547) -> (8.9249, -31.8259)
  line L220 (12.5227, -29.6823) -> (12.6506, -30.0389)
  line L221 (9.4983, -31.6681) -> (9.2972, -31.347)
  line L222 (9.6828, -34.678) -> (9.7906, -34.6098)
  line L223 (13.2638, -32.7547) -> (13.1379, -32.9981)
  line L224 (12.3236, -32.9549) -> (12.0165, -32.6685)
  line L225 (2.8001, -31.5661) -> (3.2153, -31.5661)
  spline S37 degree 3 poles (-1.6956, -31.9118) (-1.6412, -31.8385) (-1.5265, -31.7307) (-1.4407, -31.6723) knots 0 0 0 0 1 1 1 1
  line L226 (12.4958, -31.1635) -> (12.016, -31.2519)
  line L227 (8.1589, -33.674) -> (8.1589, -33.9548)
  line L228 (11.1492, -32.4066) -> (11.1726, -32.4066)
  line L229 (3.1877, -33.9981) -> (3.1877, -34.4467)
  line L230 (10.0445, -29.9848) -> (10.1836, -30.3954)
  spline S38 degree 3 poles (-2.7558, -32.5577) (-3.1344, -32.5577) (-3.1402, -32.5559) (-3.1402, -32.4397) knots 0 0 0 0 1 1 1 1
  line L231 (9.2356, -34.2806) -> (8.9924, -34.0296)
  line L232 (11.9535, -33.2323) -> (11.9535, -33.5834)
  line L233 (9.6995, -31.9892) -> (9.4983, -31.6681)
  line L234 (10.0073, -34.3507) -> (9.9514, -34.4411)
  line L235 (8.9655, -33.7304) -> (8.9387, -33.4311)
  spline S39 degree 3 poles (2.7623, -35.096) (2.4462, -34.8809) (2.4103, -34.7864) (2.3923, -34.1226) knots 0 0 0 0 1 1 1 1
  spline S40 degree 3 poles (3.153, -32.7657) (3.1685, -32.7502) (3.002, -32.5261) (2.7831, -32.2678) knots 0 0 0 0 1 1 1 1
  line L236 (1.0627, -32.3198) -> (0.012, -32.3325)
  line L237 (10.42, -30.419) -> (10.6565, -30.4425)
  line L238 (9.844, -29.5128) -> (9.8747, -29.5435)
  line L239 (11.9535, -33.5834) -> (11.9535, -33.9345)
  line L240 (-4.1083, -33.03) -> (-2.9986, -33.03)
  line L241 (9.9054, -29.5743) -> (10.0445, -29.9848)
  line L242 (9.7035, -34.9425) -> (9.5749, -34.7463)
  line L243 (8.1589, -33.3932) -> (8.1589, -33.674)
  line L244 (10.0921, -33.9288) -> (10.0073, -34.3507)
  line L245 (11.1726, -32.4066) -> (11.5631, -32.8194)
  line L246 (9.8475, -34.6086) -> (9.9045, -34.6074)
  line L247 (9.9514, -34.4411) -> (9.8955, -34.5315)
  line L248 (10.7393, -33.5887) -> (10.7393, -33.0857)
  line L249 (8.0179, -33.8106) -> (7.9664, -33.6019)
  line L250 (10.4582, -32.1018) -> (9.8665, -32.1007)
  line L251 (10.7393, -32.5827) -> (10.9326, -32.4946)
  line L252 (8.2371, -29.8221) -> (8.3172, -29.6722)
  line L253 (10.9326, -32.4946) -> (11.1259, -32.4066)
  line L254 (12.8364, -33.3909) -> (12.7143, -33.3909)
  line L255 (8.0884, -33.8827) -> (8.0179, -33.8106)
  line L256 (8.1194, -30.2975) -> (8.1569, -29.9719)
  line L257 (1.0627, -33.761) -> (1.0627, -32.3198)
  spline S41 degree 3 poles (3.0842, -31.0861) (2.4509, -31.1038) (2.3292, -31.0853) (2.1948, -30.951) knots 0 0 0 0 1 1 1 1
  line L258 (8.9924, -34.0296) -> (8.9655, -33.7304)
  line L259 (8.1282, -31.2682) -> (8.5266, -31.547)
  line L260 (13.0121, -33.2414) -> (12.8214, -33.2414)
  line L261 (-2.9986, -33.7856) -> (-4.0375, -33.7856)
  line L262 (10.7393, -33.0857) -> (10.7393, -32.5827)
  line L263 (9.8321, -35.1387) -> (9.7035, -34.9425)
  spline S42 degree 3 poles (4.4934, -35.2023) (2.9378, -35.2023) (2.9164, -35.201) (2.7623, -35.096) knots 0 0 0 0 1 1 1 1
  line L264 (8.1569, -29.9719) -> (8.2371, -29.8221)
  line L265 (10.9518, -29.5125) -> (11.3958, -29.4065)
  spline S43 degree 3 poles (2.9911, -32.7939) (3.0646, -32.7939) (3.1375, -32.7812) (3.153, -32.7657) knots 0 0 0 0 1 1 1 1
  line L266 (8.1589, -33.9548) -> (8.0884, -33.8827)
  line L267 (7.8792, -31.4141) -> (8.0358, -31.2682)
  line L268 (11.5631, -32.8194) -> (11.9535, -33.2323)
  line L269 (9.4789, -34.5315) -> (9.2356, -34.2806)
  line L270 (9.8683, -35.1387) -> (9.8321, -35.1387)
  line L271 (10.1836, -30.3954) -> (10.42, -30.419)
  line L272 (9.8955, -34.5315) -> (9.6872, -34.5315)
  line L273 (10.177, -33.507) -> (10.0921, -33.9288)
  spline S44 degree 3 poles (-1.4407, -31.6723) (-1.2882, -31.5686) (-1.2543, -31.5661) (-0.0047, -31.5661) knots 0 0 0 0 1 1 1 1
  spline S45 degree 3 poles (2.7831, -32.2678) (2.5191, -31.9564) (2.3849, -31.7591) (2.3849, -31.6821) knots 0 0 0 0 1 1 1 1
  line L274 (1.8183, -33.6273) -> (1.8183, -35.2023)
  line L275 (0.012, -32.3325) -> (-1.0388, -32.3452)
  line L276 (1.8183, -35.2023) -> (1.4405, -35.2023)
  spline S46 degree 3 poles (2.3849, -31.6821) (2.3849, -31.5676) (2.3906, -31.5661) (2.8001, -31.5661) knots 0 0 0 0 1 1 1 1
  line L277 (8.0369, -33.3932) -> (8.1589, -33.3932)
  line L278 (9.0947, -33.1275) -> (9.3638, -32.805)
  line L279 (8.9387, -33.4311) -> (9.0167, -33.2793)
  line L280 (9.5, -37.5) -> (-9.5, -37.5)
  line L281 (10, -27.5) -> (-10, -27.5)
  line L282 (0, -37.8678) -> (0, -27.1322)
  line L283 (0, -32.5) -> (0.2147, -32.5)
  spline S47 degree 3 poles (-4.1744, -31.5661) (-2.9513, -31.566) (-2.9144, -31.5687) (-2.7628, -31.6718) knots 0 0 0 0 0.998349 0.998349 0.998349 0.998349
  line L284 (-2.762, -31.6723) -> (-2.7628, -31.6718)
  constraint coincident L131.start L158.end
  constraint midpoint L282 L283.start
emboss "Gravure en relief3" depth 0.3 profiles "Esquisse9" section 1 onto face at (9.9503, -30.6667, -100.9957) on bodies 7 bodies 7
pattern_circular "Réseau C1" count 3 over 360 about axis through (0, -37.5, -100) along (0, 1, 0) of "Gravure en relief3"
sketch "Esquisse10" plane through (0, -27.5, 0) normal (0, 1, 0) x (-1, 0, 0)
  circle A0 centre (0, -100) radius 10
  circle A1 centre (0, -100) radius 4.5
  dimension "d121" = 9
  constraint concentric A0 A1
  measures "d121" diameter of A1
extrude "Extrusion20" cut sketch "Esquisse10" against normal blind 8 contours A1 bodies 7
hidden bodies 1 2 5 6
